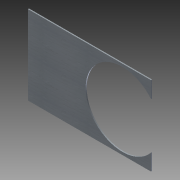
# Autodesk Inventor part: Fore_Top
Saved by Autodesk Inventor 2011 SP1 (Build 150282100, 282)
## iProperties
Created: 2011-05-30
Part Number: Fore_Top
Document SubType Name: Modeling
Designer: Andrew G. Meyer
Mass: 152.183 g
Surface Area: 1008.08 cm^2
Volume: 152.183 cm^3
Density: 1 g/cm^3
Author: Andrew G. Meyer
Autodesk Inventor part; units mm, degrees
ref_plane "YZ Plane" through (0, 0, 0) normal (1, 0, 0) x (0, 1, 0)
ref_plane "XZ Plane" through (0, 0, 0) normal (0, 1, 0) x (-1, 0, 0)
ref_plane "XY Plane" through (0, 0, 0) normal (0, 0, 1) x (1, 0, 0)
sketch "Sketch1" plane through (0, 0, 0) normal (0, 0, 1) x (1, 0, 0)
  line L0 (-152.4, 114.3) -> (203.2, 114.3)
  line L1 (203.2, 114.3) -> (203.2, -114.3)
  line L2 (203.2, -114.3) -> (-152.4, -114.3)
  line L3 (-152.4, -114.3) -> (-152.4, 114.3)
  point P0 (0, 0)
  dimension "d0" = 355.6
  dimension "d1" = 228.6
  dimension "d2" = 114.3
  dimension "d3" = 152.4
  constraints: 8 end point, 2 parallel, 1 horizontal, 1 perpendicular
  measures "d0" distance of L0.start L0.end
  measures "d1" distance of L2.end L0.start
  measures "d2" distance from line of L0 point (0, 0)
  measures "d3" distance from line of L3 point (0, 0)
extrude "Extrusion1" add sketch "Sketch1" against normal blind 3.175
hole "Hole1" at (120.65, 0, 0) direction (0, 0, -1) diameter 212.725 depth 3.175 tip angle 118
body "Solid1"
